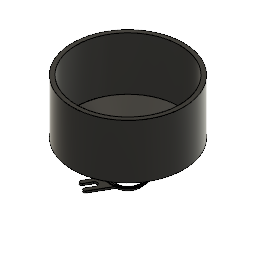
HeadplateShield2P v1 (Autodesk Fusion 360 design; units mm, degrees)
Autodesk Fusion 360 part; units mm, degrees
sketch "Sketch1" plane through (0, 0, 0) normal (1, 0, 0) x (0, 0, -1)
  line L0 (-74.3554, -0.45) -> (-74.3554, 10.5) construction
  line L1 (-70.1054, 0.0307) -> (-69.8554, 0.0307)
  line L2 (-68.3554, 2.2807) -> (-68.3554, 2.5307)
  line L3 (-68.3554, 2.5307) -> (-67.8554, 2.5307)
  line L4 (-67.8554, 2.5307) -> (-67.8554, 2.2807)
  line L5 (-69.8554, 1.5463) -> (-68.3554, 2.2807)
  arc A0 (-69.8554, 1.5463) -> (-70.1054, 0.0307) centre (-69.4408, 0.6995) ccw
  line L6 (-68.3554, 2.2807) -> (-67.8554, 2.2807) construction
  arc A1 (-68.0001, 2.0486) -> (-67.8554, 2.2807) centre (-68.1137, 2.2807) ccw
  arc A2 (-69.0442, 1.3643) -> (-69.8554, 0.0307) centre (-68.8453, 0.3299) ccw
  arc A3 (-69.0442, 1.3643) -> (-68.8168, 1.5791) centre (-69.0992, 1.6505) ccw
  arc A4 (-68.7229, 1.6948) -> (-68.8168, 1.5791) centre (-68.645, 1.5356) ccw
  line L7 (-68.7229, 1.6948) -> (-68.0001, 2.0486)
  dimension "d52" = 4.5
  dimension "d55" = 6
  dimension "d56" = 6.5
  dimension "d59" = 4.5
  dimension "d79" = 4.25
  dimension "d81" = 0.25
  dimension "d83" = 2.25
  constraint perpendicular L0 L1
  constraint perpendicular L2 L3
  constraint tangent L5 A0
  constraint perpendicular L3 L4
  constraint perpendicular L4 L6
  constraint horizontal L3
  constraint tangent L4 A1
  constraint tangent A2 A3
  constraint tangent A4 L7
  constraint tangent A1 L7
  constraint parallel L5 L7
  constraint tangent A3 A4
  measures "d52" distance of L0 L1.end
  measures "d55" distance of L0 L2.start
  measures "d56" distance of L0 L4.end
  measures "d59" distance of L0 L5.start
  measures "d79" distance of L0 L1.start
  measures "d81" distance of L3 L6
  measures "d83" distance of L1 L6
revolve "Revolve1" add sketch "Sketch1" angle 360 about axis through (0, -0.45, 74.3554) along (0, 1, 0) makes body 1
copy_body "Body->Comp1" bodies 1 removing the originals makes body 2 in component "Headplate"
sketch "Sketch1 (2)" plane through (0, 0, 0) normal (1, 0, 0) x (0, 0, -1) in component "2p Sleeve"
  line L0 (-80.8554, 2.5307) -> (-67.8554, 2.5307) construction
  line L1 (-94.8554, 13.8531) -> (-94.8554, 33.8531)
  line L2 (-94.8554, 33.8531) -> (-93.3554, 33.8531)
  line L3 (-80.8554, 9.2531) -> (-83.3554, 9.2531)
  line L4 (-83.3554, 9.2531) -> (-94.8554, 13.8531)
  line L5 (-80.8554, 9.2531) -> (-93.3554, 14.2531)
  line L6 (-93.3554, 33.8531) -> (-93.3554, 14.2531)
  line L7 (-81.8554, 9.2531) -> (-82.6054, 9.2531) construction
  line L8 (-82.6054, 9.2531) -> (-82.6054, 8.2531)
  line L9 (-82.6054, 8.2531) -> (-81.8554, 8.2531)
  line L10 (-81.8554, 8.2531) -> (-81.8554, 9.2531)
  line L11 (-74.3554, 0.0307) -> (-74.3554, 62.8357)
  line L12 (-78.8554, 0.0307) -> (-69.8554, 0.0307)
  circle A0 through (-78.6054, 0.0307, 0) (-72.2304, 0.0307, 3.6806) (-72.2304, 0.0307, -3.6806)
  point P0 (-74.3554, 0.0307)
  dimension "d125" = 20
  dimension "d127" = 2.5
  dimension "d135" = 1
  dimension "d138" = 0.75
  dimension "d139" = 1.5
  dimension "d140" = 1
  dimension "d142" = 13
  dimension "d144" = 5
  dimension "d183" = 38
  constraint perpendicular L2 L6
  constraint parallel L4 L5
  constraint vertical L6
  constraint vertical L1
  constraint horizontal L7
  constraint vertical L8
  constraint horizontal L9
  constraint vertical L10
  constraint coincident L3 L7.start
  constraint perpendicular L0 L11
  constraint horizontal L3
  constraint coincident P0 L11.start
  measures "d125" distance of L1.start L1.end
  measures "d127" distance of L3.start L3.end
  measures "d135" distance of L3.start L10
  measures "d138" distance of L8.end L9.end
  measures "d139" distance of L2.end L1.end
  measures "d140" distance of L7.end L8.end
  measures "d144" distance of L3 L5.end
revolve "Revolve1'" add sketch "Sketch1 (2)" angle 360 about axis through (0, 0.0307, 74.3554) along (0, 1, 0) separate body makes body 3 in component "2p Sleeve"
sketch "Sketch1 (3)" plane through (0, 0.0307, 0) normal (0, -1, 0) x (1, 0, 0) in component "Headplate"
  circle A0 centre (0, 74.3554) radius 4.5
  circle A1 centre (0, 74.3554) radius 4.25
  line L0 (-8.1651, 65.2131) -> (-0.2942, 78.8458)
  line L1 (0, 74.3554) -> (0, 54.3551)
  line L2 (0, 74.3554) -> (-10, 57.0349) construction
  line L3 (0, 74.3554) -> (-10, 74.3554)
  line L4 (-5.366, 67.0612) -> (-6.866, 64.4631)
  arc A2 (-4, 67.4272) -> (-5.366, 67.0612) centre (-4.5, 66.5612) ccw
  line L5 (-3.8349, 62.7131) -> (4.0359, 76.3458)
  line L6 (-3.634, 66.0612) -> (-5.134, 63.4631)
  arc A3 (-3.634, 66.0612) -> (-4, 67.4272) centre (-4.5, 66.5612) ccw
  arc A4 (-8.1651, 65.2131) -> (-6.866, 64.4631) centre (-7.5155, 64.8381) ccw
  arc A5 (-5.134, 63.4631) -> (-3.8349, 62.7131) centre (-4.4845, 63.0881) ccw
  line L7 (-7.5155, 64.8381) -> (-6, 63.9631) construction
  line L8 (-5.4151, 69.9762) -> (-1.0849, 67.4762)
  point P0 (-4.5, 66.5612)
  dimension "d157" = 30
  dimension "d159" = 2.5
  dimension "d161" = 9
  dimension "d162" = 2
  dimension "d172" = 0.75
  dimension "d178" = 12
  dimension "d186" = 5.5
  constraint coincident A0.centre A1.centre
  constraint vertical L1
  constraint coincident A0 L0.end
  constraint coincident L2 P0
  constraint parallel L0 L2
  constraint perpendicular L1 L3
  constraint coincident P0 A2.centre
  constraint parallel L0 L4
  constraint tangent L4 A2
  constraint coincident L2 A2.start
  constraint symmetric L0.end L2 L5.end
  constraint symmetric L2 L4.start L6.start
  constraint symmetric L2 L0.start L5.start
  constraint symmetric L2 L4.end L6.end
  constraint symmetric L2 A2 A3
  constraint symmetric L2 A2.start A3.end
  constraint symmetric L2 A4 A5
  constraint coincident A4.centre L7.start
  constraint coincident L2 L7.end
  constraint perpendicular L2 L7
  constraint coincident L0 L8.start
  constraint coincident L5 L8.end
  constraint perpendicular L5 L8
  measures "d157" angle of L1 L2
  measures "d159" distance of L0 L2
  measures "d161" distance of A0.centre P0
  measures "d162" diameter of A2
  measures "d172" radius of A4
  measures "d178" distance of A0.centre L7
  measures "d186" distance of A4.centre L8
ref_plane "WorkPlane1" through (-5, 0.0307, 74.3554) normal (0, 0, 1) x (-1, 0, 0) in component "Headplate"
extrude "Extrude2" add sketch "Sketch1 (3)" against normal blind 0.75 separate body contours L0 L4 A2 L5 L6 A3 A4 A5 L8 makes body 4 in component "Headplate"
extrude "Extrude3" add 1 faces at (-3.9717, 0.5307, 69.1429) along direction (0.5, 0, 0.866025) up to near side of body 2 on bodies 4 bodies 4 2 in component "Headplate"
mirror "Mirror2" about plane through (-5, 0.0307, 74.3554) normal (0, 0, 1) of bodies 4 merged in component "Headplate"
component "2p Sleeve" placed x (1, 0, 0) y (0, 1, 0) z (0, 0, 1) at (0, 0, 0)
component "Headplate" placed x (1, 0, 0) y (0, 1, 0) z (0, 0, 1) at (0, 0, 0)
equation "d52 = bottomOuterDiameter * 0.5"
equation "d55 = topInnerDiameter * 0.5"
equation "d56 = topOuterDiameter * 0.5"
equation "d59 = middleInnerDiameter * 0.5"
equation "d79 = bottomInnerDiameter * 0.5"
equation "d81 = topLipHeight"
equation "d83 = totalHeight - topLipHeight"
equation "d125 = sleeveHeight"
equation "d127 = sleeveBottomDiameter"
equation "d135 = maxToleranceSleeve"
equation "d138 = sleeveMaxPlateLipWidth"
equation "d139 = wallThickness"
equation "d140 = sleevePlateLipHeight"
equation "d142 = topOuterDiameter"
equation "d144 = objectiveTaperLength"
equation "d157 = holderMaxAngle"
equation "d159 = holderMaxWidth * 0.5"
equation "d161 = holderOpeningFromCenter"
equation "d162 = holderOpeningDiameter"
equation "d172 = holderProngWidth * 0.5"
equation "d174 = -holderMaxHeight"
equation "d178 = holderLengthFromCenter"
equation "d183 = objectiveDiameter"
equation "d186 = holderLengthFromCenter - topOuterDiameter * 0.5"
equation "bottomInnerDiameter = 8.5 mm"
equation "bottomOuterDiameter = 9 mm"
equation "topInnerDiameter = 12 mm"
equation "topOuterDiameter = 13 mm"
equation "middleInnerDiameter = 9 mm"
equation "totalHeight = 2.5 mm"
equation "topLipHeight = 0.25 mm"
equation "holderLengthFromCenter = 12 mm"
equation "holderWidth = 5 mm"
equation "holderOpeningDiameter = 2 mm"
equation "holderOpeningFromCenter = 9 mm"
equation "holderHeight = 0.75 mm"
equation "holderAngle = 30 deg"
equation "holderProngWidth = ( holderMaxWidth - holderOpeningDiameter ) * 0.5"
equation "wallThickness = 1.5 mm"
equation "objectiveDiameter = 38 mm"
equation "sleeveHeight = 20 mm"
equation "toleranceSleeve = 1 mm"
equation "objectiveTaperLength = 5 mm"
equation "sleeveBottomDiameter = 2.5 mm"
equation "sleevePlateLipWidth = 0.75 mm"
equation "sleevePlateLipHeight = 1 mm"
equation "holderMaxAngle = max(0 deg; min(89.99 deg; holderAngle))"
equation "holderMaxHeight = max(0.25 mm; min(totalHeight - topLipHeight; holderHeight))"
equation "holderMaxWidth = max(( holderOpeningDiameter + 1 mm ); min(bottomOuterDiameter; holderWidth))"
equation "maxToleranceSleeve = max(0.1 mm; min(sleeveBottomDiameter - sleevePlateLipWidth; toleranceSleeve))"
equation "sleeveMaxPlateLipWidth = max(0.5 mm; min(sleeveBottomDiameter - ( sleevePlateLipWidth + maxToleranceSleeve ); sleevePlateLipWidth))"
